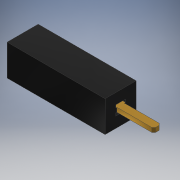
# Autodesk Inventor part: CON-HEM
Saved by Autodesk Inventor 2018.3 (Build 223284000, 284)
## iProperties
Created: 2020-10-22
Part Number: CON-HEM
Material: Genérico
Document SubType Name: Modeling
Designer: laguerre
Density: 8.47 g/cm^3
Appearance: Suave - Negro
Author: laguerre
Autodesk Inventor part; units mm, degrees
ref_plane "YZ Plane" through (0, 0, 0) normal (1, 0, 0) x (0, 1, 0)
ref_plane "XZ Plane" through (0, 0, 0) normal (0, 1, 0) x (-1, 0, 0)
ref_plane "XY Plane" through (0, 0, 0) normal (0, 0, 1) x (1, 0, 0)
sketch "Boceto39" plane through (0, 0, 0) normal (0, 0, 1) x (1, 0, 0)
  line L0 (-1.27, 1.27) -> (1.27, 1.27)
  line L1 (1.27, 1.27) -> (1.27, -1.27)
  line L2 (1.27, -1.27) -> (-1.27, -1.27)
  line L3 (-1.27, -1.27) -> (-1.27, 1.27)
  point P0 (0, 0)
  point P1 (0, 1.27)
  point P2 (-1.27, 0)
  dimension "d373" = 2.54
  constraints: 8 end point, 2 midpoint, 2 parallel, 2 perpendicular, 1 horizontal, 1 horizontal alignment, 1 vertical alignment
  measures "d373" distance of L0.end L1.end
extrude "Extrusión13" add sketch "Boceto39" along normal blind 8
sketch "Boceto40" plane through (0, 0, 8) normal (0, 0, 1) x (1, 0, 0)
  line L0 (-0.4, 0.4) -> (0.4, 0.4)
  line L1 (0.4, 0.4) -> (0.4, -0.4)
  line L2 (0.4, -0.4) -> (-0.4, -0.4)
  line L3 (-0.4, -0.4) -> (-0.4, 0.4)
  point P0 (0, 0)
  point P1 (0, 0.4)
  point P2 (-0.4, 0)
  dimension "d376" = 0.8
  constraints: 8 end point, 2 midpoint, 2 parallel, 2 perpendicular, 1 horizontal, 1 horizontal alignment, 1 vertical alignment
  measures "d376" distance of L0.start L0.end
extrude "Extrusión14" cut sketch "Boceto40" against normal blind 8
chamfer "Chaflán5" distance 0.3 angle 45 4 edges at (0, 0.4, 8) (0.4, 0, 8) (0, -0.4, 8) (-0.4, 0, 8)
sketch "Boceto42" plane through (0, 0, 0) normal (0, 1, 0) x (-1, 0, 0)
  line L0 (-0.4, 7.7) -> (-0.4, 0) construction
  line L1 (0.4, 7.7) -> (0.4, 0) construction
  line L2 (-0.4, 0) -> (-0.3, 0)
  line L3 (-1.27, 0) -> (1.27, 0) construction
  line L4 (-0.3, -3) -> (-0.3, 0)
  line L5 (0.3, -3) -> (-0.3, -3)
  line L6 (0.3, -3) -> (0.3, 0)
  line L7 (0.3, 0) -> (0.4, 0)
  line L8 (0.4, 0) -> (0.4, 0.3601)
  line L9 (0.4, 0.3601) -> (-0.4, 0.3601)
  line L10 (-0.4, 0.3601) -> (-0.4, 0)
  point P0 (0, 0)
  point P1 (0, -3)
  point P2 (0, 0)
  dimension "d386" = 0.6
  dimension "d387" = 3
  constraints: 16 end point, 6 perpendicular, 4 point on line, 2 midpoint, 1 vertical alignment
  measures "d386" distance of L5.start L4.start
  measures "d387" distance of L5.start L6.end
extrude "Extrusión16" add sketch "Boceto42" along normal mid plane 0.35
chamfer "Chaflán6" distance 0.15 angle 45 2 edges at (0.3, 0, -3) (-0.3, 0, -3)
